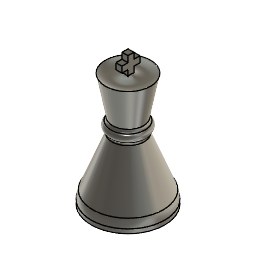
roi (Autodesk Fusion 360 design; units mm, degrees)
part number: 2026-06-29-13-41-10-715
Autodesk Fusion 360 part; units mm, degrees
note: some values were not read from the file. Set by a fixed rule: which sketch regions a step uses.
sketch "Esquisse1" plane through (0, 0, 0) normal (0, 1, 0) x (1, 0, 0)
  line L0 (0, 0) -> (13, 0)
  line L1 (13, 0) -> (0, 0)
  line L2 (0, 0) -> (0, -42)
  line L3 (13, 0) -> (13, -3)
  line L4 (8, -40) -> (5.3072, -25.7485)
  line L5 (13, -3) -> (5.3072, -22.8015)
  circle A0 centre (5.3072, -24.275) radius 1.4735
  line L6 (5.3072, -25.7485) -> (5.3072, -22.8015)
  line L7 (0, -42) -> (-0.7188, -42)
  arc A1 (8, -40) -> (-0.7188, -42) centre (4.75, -45.8363) ccw
  line L8 (0, 0) -> (4.1, 0)
  line L9 (4.1, 0) -> (4.1, -3.2)
  line L10 (4.1, -3.2) -> (0, -3.2)
  line L11 (0, -3.2) -> (0, 0)
  dimension "d1" = 13
  dimension "d2" = 42
  dimension "d3" = 3
  dimension "d4" = 4.1
  dimension "d5" = 3.2
  constraint coincident L0.start L1.end
  constraint horizontal L0
  constraint perpendicular L1 L2
  constraint perpendicular L0 L3
  constraint coincident L5.end A0
  constraint coincident L4.end A0
  constraint vertical L6
  constraint perpendicular L2 L7
  constraint horizontal L8
  constraint vertical L9
  constraint horizontal L10
  constraint vertical L11
  constraint midpoint A0.centre L6
  measures "d1" distance of L0.start L0.end
  measures "d2" distance of L0.start L2.end
  measures "d3" distance of L0.end L3.end
  measures "d4" distance of L9.end L10.end
  measures "d5" distance of L8.end L9.end
revolve "Révolution1" add sketch "Esquisse1" angle 360 about axis through (0, 0, 0) along (0, 0, 1) contours L0 L1 L2 L3 L4 L5 A0 A1 L9 L10 | A0 L6 | A0 L6
fillet "Congé1" radius 1 2 edges at (-4.9481, -1.9192, 25.7485) (-4.9481, -1.9192, 22.8015)
fillet "Congé2" radius 8 1 edges at (-12.1203, -4.701, 3)
sketch "Esquisse2" plane through (0, 0, 0) normal (1, 0, 0) x (0, 1, 0)
  line L0 (-1.07, 40) -> (-1.07, 42.14)
  line L1 (-1.07, 42.14) -> (-3.21, 42.14)
  line L2 (-3.21, 42.14) -> (-3.21, 44.28)
  line L3 (-3.21, 44.28) -> (-1.07, 44.28)
  line L4 (-1.07, 44.28) -> (-1.07, 46.42)
  line L5 (-1.07, 46.42) -> (1.07, 46.42)
  line L6 (1.07, 46.42) -> (1.07, 44.28)
  line L7 (1.07, 44.28) -> (3.21, 44.28)
  line L8 (3.21, 44.28) -> (3.21, 42.14)
  line L9 (3.21, 42.14) -> (1.07, 42.14)
  line L10 (1.07, 42.14) -> (1.07, 40)
  line L11 (1.07, 40) -> (-1.07, 40)
  point P0 (0, 40)
  point P1 (0, 40)
  dimension "d12" = 2.14
  constraint vertical L0
  constraint perpendicular L0 L1
  constraint perpendicular L1 L2
  constraint perpendicular L0 L3
  constraint perpendicular L1 L4
  constraint horizontal L5
  constraint perpendicular L5 L6
  constraint parallel L5 L9
  constraint perpendicular L9 L10
  constraint horizontal L11
  constraint vertical L8
  constraint horizontal L7
  constraint midpoint L11 P1
  constraint coincident P1 P0
  constraint collinear L0 L4
  constraint collinear L6 L10
  constraint collinear L3 L7
  constraint collinear L1 L9
  constraint equal L2 L3
  constraint equal L4 L5
  constraint equal L6 L7
  constraint equal L8 L9
  constraint equal L9 L10
  measures "d12" distance of L0.start L10.end
extrude "Extrusion1" add sketch "Esquisse2" along normal blind 2.12 from surface at -1.06
